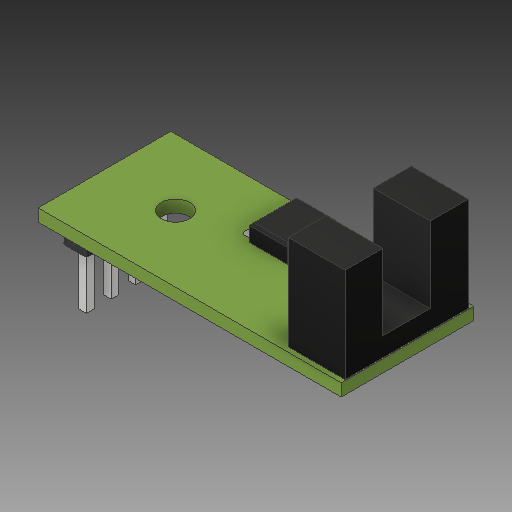
# Autodesk Inventor part: Оптический датчик
Saved by Autodesk Inventor 2019 (Build 230136000, 136)
## iProperties
Created: 2019-08-06
Part Number: Оптический датчик
Material: Типовые
Document SubType Name: Modeling
Designer: user
Density: 1 g/cm^3
Appearance: По умолчанию
Mass: 1.23373 g
Surface Area: 15.9477 cm^2
Volume: 1.23373 cm^3
Author: user
Autodesk Inventor part; units mm, degrees
ref_plane "YZ Plane" through (0, 0, 0) normal (1, 0, 0) x (0, 1, 0)
ref_plane "XZ Plane" through (0, 0, 0) normal (0, 1, 0) x (-1, 0, 0)
ref_plane "XY Plane" through (0, 0, 0) normal (0, 0, 1) x (1, 0, 0)
sketch "Эскиз1" plane through (0, 0, 0) normal (0, 1, 0) x (-1, 0, 0)
  line L0 (-16, 7) -> (16, 7)
  line L1 (16, 7) -> (16, -7)
  line L2 (16, -7) -> (-16, -7)
  line L3 (-16, -7) -> (-16, 7)
  line L4 (-16, 7) -> (16, -7) construction
  line L5 (16, 7) -> (-16, -7) construction
  point P0 (0, 0)
  dimension "d0" = 32
  dimension "d1" = 14
  constraints: 12 end point, 2 midpoint, 2 parallel, 1 horizontal, 1 perpendicular
  measures "d0" distance of L1.end L2.end
  measures "d1" distance of L0.end L1.end
extrude "Выдавливание1" add sketch "Эскиз1" along normal blind 1.3
sketch "Эскиз4" plane through (0, 1.3, 0) normal (0, 1, 0) x (1, 0, 0)
  line L0 (-16, -7) -> (16, -7) projected
  line L1 (16, -7) -> (16, -6.5)
  line L2 (16, -7) -> (16, 7) projected
  line L3 (16, -6.5) -> (15.9, -6.5)
  line L4 (15.9, -6.5) -> (9.9, -6.5)
  line L5 (9.9, -6.5) -> (9.9, 6.5)
  line L6 (9.9, 6.5) -> (15.9, 6.5)
  line L7 (15.9, 6.5) -> (15.9, -6.5)
  point P0 (0, 0)
  dimension "d13" = 0.5
  dimension "d14" = 0.1
  dimension "d15" = 6
  dimension "d16" = 13
  constraints: 12 end point, 2 parallel, 2 perpendicular, 1 horizontal, 1 point on line
  measures "d13" distance of L0.end L1.end
  measures "d14" distance of L1.end L3.end
  measures "d15" distance of L5.end L6.end
  measures "d16" distance of L4.end L5.end
extrude "Выдавливание4" add sketch "Эскиз4" along normal blind 10
sketch "Эскиз5" plane through (0, 11.3, 0) normal (0, 1, 0) x (1, 0, 0)
  line L0 (9.9, 6.5) -> (9.9, -6.5) projected
  line L1 (15.9, -2.5) -> (9.9, -2.5)
  line L2 (9.9, -2.5) -> (9.9, 2.5)
  line L3 (9.9, 2.5) -> (15.9, 2.5)
  line L4 (15.9, 2.5) -> (15.9, -2.5)
  line L5 (15.9, -2.5) -> (9.9, 2.5) construction
  line L6 (9.9, -2.5) -> (15.9, 2.5) construction
  point P0 (0, 0)
  point P1 (12.9, 0)
  dimension "d19" = 5
  constraints: 12 end point, 2 midpoint, 2 parallel, 1 horizontal, 1 perpendicular, 1 point on line
  measures "d19" distance of L1.end L2.end
extrude "Выдавливание5" cut sketch "Эскиз5" against normal blind 8
sketch "Эскиз6" plane through (0, 1.3, 0) normal (0, 1, 0) x (1, 0, 0)
  line L0 (-16, 7) -> (-16, -7) projected
  line L1 (-16, 0) -> (-10, 0)
  line L2 (-10, 0) -> (-7, 0)
  circle A0 centre (-8.5, 0) radius 1.5
  point P0 (0, 0)
  dimension "d22" = 6
  dimension "d23" = 3
  constraints: 4 end point, 2 midpoint, 1 horizontal, 1 horizontal alignment, 1 point on line, 2 other
  measures "d22" distance of L1.start L1.end
  measures "d23" distance of L1.end L2.end
extrude "Выдавливание6" cut sketch "Эскиз6" against normal blind 8
sketch "Эскиз10" plane through (0, 1.3, 0) normal (0, 1, 0) x (1, 0, 0)
  line L0 (2.3, 6) -> (-1.7, 6)
  line L1 (-1.7, 6) -> (-1.7, 1)
  line L2 (-1.7, 1) -> (2.3, 1)
  line L3 (2.3, 1) -> (2.3, 6)
  line L4 (-12.7, 2.9) -> (-12.7, 4.9) projected
  line L5 (16, 7) -> (-16, 7) projected
  point P0 (0, 0)
  dimension "d49" = 4
  dimension "d50" = 5
  dimension "d51" = 11
  dimension "d52" = 1
  constraints: 8 end point, 2 parallel, 1 horizontal, 1 perpendicular
  measures "d49" distance of L2.end L1.end
  measures "d50" distance of L1.end L0.end
  measures "d51" distance between parallel lines of L4 L1
  measures "d52" distance between parallel lines of L5 L0
extrude "Выдавливание9" add sketch "Эскиз10" along normal blind 1.8
chamfer "Фаска1" distance 0.25 angle 45 4 edges at (-1.7, 3.1, -3.5) (0.3, 3.1, -1) (2.3, 3.1, -3.5) (0.3, 3.1, -6)
sketch "Эскиз11" plane through (0, 1.3, 0) normal (0, 1, 0) x (1, 0, 0)
  line L0 (-1.7, 1) -> (-1.7, 6) projected
  line L1 (-1.7, 6) -> (-1.7, 5.8)
  line L2 (-1.7, 5.8) -> (-2.7, 5.8)
  line L3 (-2.7, 5.8) -> (-2.7, 5.3)
  line L4 (-2.7, 5.3) -> (-1.7, 5.3)
  line L5 (-1.7, 5.3) -> (-1.7, 5.8)
  line L6 (-1.7, 4.7) -> (-1.7, 4.5)
  line L7 (-1.7, 4.5) -> (-2.7, 4.5)
  line L8 (-2.7, 4.5) -> (-2.7, 4)
  line L9 (-2.7, 4) -> (-1.7, 4)
  line L10 (-1.7, 4) -> (-1.7, 4.5)
  line L11 (-1.7, 3.4) -> (-1.7, 3.2)
  line L12 (-1.7, 3.2) -> (-2.7, 3.2)
  line L13 (-2.7, 3.2) -> (-2.7, 2.7)
  line L14 (-2.7, 2.7) -> (-1.7, 2.7)
  line L15 (-1.7, 2.7) -> (-1.7, 3.2)
  line L16 (-1.7, 2.1) -> (-1.7, 1.9)
  line L17 (-1.7, 1.9) -> (-2.7, 1.9)
  line L18 (-2.7, 1.9) -> (-2.7, 1.4)
  line L19 (-2.7, 1.4) -> (-1.7, 1.4)
  line L20 (-1.7, 1.4) -> (-1.7, 1.9)
  line L21 (-1.7, 6) -> (2.3, 6) projected
  line L22 (0.3, 6) -> (0.3, 4.6)
  line L23 (2.3, 1) -> (2.3, 6)
  line L24 (2.3, 6) -> (2.3, 5.8)
  line L25 (2.3, 5.8) -> (3.3, 5.8)
  line L26 (3.3, 5.8) -> (3.3, 5.3)
  line L27 (3.3, 5.3) -> (2.3, 5.3)
  line L28 (2.3, 5.3) -> (2.3, 5.8)
  line L29 (2.3, 4.7) -> (2.3, 4.5)
  line L30 (2.3, 4.5) -> (3.3, 4.5)
  line L31 (3.3, 4.5) -> (3.3, 4)
  line L32 (3.3, 4) -> (2.3, 4)
  line L33 (2.3, 4) -> (2.3, 4.5)
  line L34 (2.3, 3.4) -> (2.3, 3.2)
  line L35 (2.3, 3.2) -> (3.3, 3.2)
  line L36 (3.3, 3.2) -> (3.3, 2.7)
  line L37 (3.3, 2.7) -> (2.3, 2.7)
  line L38 (2.3, 2.7) -> (2.3, 3.2)
  line L39 (2.3, 2.1) -> (2.3, 1.9)
  line L40 (2.3, 1.9) -> (3.3, 1.9)
  line L41 (3.3, 1.9) -> (3.3, 1.4)
  line L42 (3.3, 1.4) -> (2.3, 1.4)
  line L43 (2.3, 1.4) -> (2.3, 1.9)
  point P0 (0, 0)
  dimension "d58" = 0.2
  dimension "d59" = 1
  dimension "d60" = 0.5
  dimension "d63" = 1.3
  constraints: 84 end point, 20 symmetric about line, 2 parallel, 2 point on line, 2 vertical, 1 horizontal, 1 midpoint, 1 perpendicular, 30 other
  measures "d58" distance of L0.end L1.end
  measures "d59" distance of L4.end L3.end
  measures "d60" distance of L3.end L2.end
  measures "d63" distance of L1.end L6.end
extrude "Выдавливание10" add sketch "Эскиз11" along normal blind 1
chamfer "Фаска2" distance 0.75 angle 45 8 edges at (-2.7, 2.3, -5.55) (-2.7, 2.3, -4.25) (-2.7, 2.3, -2.95) (-2.7, 2.3, -1.65) (3.3, 2.3, -1.65) (3.3, 2.3, -2.95) (3.3, 2.3, -4.25) (3.3, 2.3, -5.55)
sketch "Эскиз18" plane through (0, 0, 0) normal (0, -1, 0) x (1, 0, 0)
  line L0 (16, 7) -> (-16, 7) projected
  line L1 (-16, 7) -> (-15.3, 7)
  line L2 (-15.3, 7) -> (-15.3, 5.2)
  line L3 (-15, 5.2) -> (-13, 5.2)
  line L4 (-12.7, 4.9) -> (-12.7, 2.9)
  line L5 (-13, 2.6) -> (-15, 2.6)
  line L6 (-15.3, 2.9) -> (-15.3, 4.9)
  arc A0 (-12.7, 4.9) -> (-13, 5.2) centre (-13, 4.9) ccw
  arc A1 (-13, 2.6) -> (-12.7, 2.9) centre (-13, 2.9) ccw
  arc A2 (-15.3, 2.9) -> (-15, 2.6) centre (-15, 2.9) ccw
  arc A3 (-15, 5.2) -> (-15.3, 4.9) centre (-15, 4.9) ccw
  line L7 (-15.3, 4.4) -> (-15.3, 2.6)
  arc A4 (-15, 2.6) -> (-15.3, 2.3) centre (-15, 2.3) ccw
  line L8 (-15, 2.6) -> (-13, 2.6)
  arc A5 (-12.7, 2.3) -> (-13, 2.6) centre (-13, 2.3) ccw
  line L9 (-15.3, 0.3) -> (-15.3, 2.3)
  arc A6 (-15.3, 0.3) -> (-15, 0) centre (-15, 0.3) ccw
  line L10 (-12.7, 2.3) -> (-12.7, 0.3)
  arc A7 (-13, 0) -> (-12.7, 0.3) centre (-13, 0.3) ccw
  line L11 (-13, 0) -> (-15, 0)
  line L12 (-15.3, 1.8) -> (-15.3, 0)
  arc A8 (-15, 0) -> (-15.3, -0.3) centre (-15, -0.3) ccw
  line L13 (-15, 0) -> (-13, 0)
  arc A9 (-12.7, -0.3) -> (-13, 0) centre (-13, -0.3) ccw
  line L14 (-15.3, -2.3) -> (-15.3, -0.3)
  arc A10 (-15.3, -2.3) -> (-15, -2.6) centre (-15, -2.3) ccw
  line L15 (-12.7, -0.3) -> (-12.7, -2.3)
  arc A11 (-13, -2.6) -> (-12.7, -2.3) centre (-13, -2.3) ccw
  line L16 (-13, -2.6) -> (-15, -2.6)
  line L17 (-15.3, -0.8) -> (-15.3, -2.6)
  arc A12 (-15, -2.6) -> (-15.3, -2.9) centre (-15, -2.9) ccw
  line L18 (-15, -2.6) -> (-13, -2.6)
  arc A13 (-12.7, -2.9) -> (-13, -2.6) centre (-13, -2.9) ccw
  line L19 (-15.3, -4.9) -> (-15.3, -2.9)
  arc A14 (-15.3, -4.9) -> (-15, -5.2) centre (-15, -4.9) ccw
  line L20 (-12.7, -2.9) -> (-12.7, -4.9)
  arc A15 (-13, -5.2) -> (-12.7, -4.9) centre (-13, -4.9) ccw
  line L21 (-13, -5.2) -> (-15, -5.2)
  point P0 (0, 0)
  point P1 (-12.7, 2.6)
  point P2 (-12.7, 5.2)
  point P3 (-12.7, 2.6)
  point P4 (-12.7, 0)
  point P5 (-12.7, 0)
  point P6 (-12.7, -2.6)
  point P7 (-12.7, -2.6)
  point P8 (-15.3, -5.2)
  point P9 (-12.7, -5.2)
  dimension "d105" = 0.7
  dimension "d106" = 1.8
  dimension "d107" = 2.6
  dimension "d108" = 2.6
  dimension "d109" = 0.3
  dimension "d112" = 2.6
  constraints: 42 end point, 33 point on line, 32 point on circle, 16 centre point, 8 tangent, 3 equal radius, 2 parallel, 2 vertical, 1 collinear, 1 horizontal, 1 perpendicular, 77 other
  measures "d105" distance of L0.end L1.end
  measures "d106" distance of L1.end L2.end
  measures "d107" distance of point (-12.7, 2.6) point (-15.3, 2.6)
  measures "d108" distance of point (-12.7, 5.2) point (-12.7, 2.6)
  measures "d109" radius of A0
  measures "d112" distance of L6.start L9.start
extrude "Выдавливание11" add sketch "Эскиз18" along normal blind 2.5
sketch "Эскиз19" plane through (0, -2.5, 0) normal (0, -1, 0) x (1, 0, 0)
  line L0 (-15, 5.2) -> (-13, 5.2) projected
  line L1 (-14, 5.2) -> (-14, 3.9)
  line L2 (-14.4, 3.5) -> (-13.6, 3.5)
  line L3 (-13.6, 3.5) -> (-13.6, 4.3)
  line L4 (-13.6, 4.3) -> (-14.4, 4.3)
  line L5 (-14.4, 4.3) -> (-14.4, 3.5)
  line L6 (-14.4, 3.5) -> (-13.6, 4.3) construction
  line L7 (-13.6, 3.5) -> (-14.4, 4.3) construction
  line L8 (-14.4, 0.9) -> (-13.6, 0.9)
  line L9 (-13.6, 0.9) -> (-13.6, 1.7)
  line L10 (-13.6, 1.7) -> (-14.4, 1.7)
  line L11 (-14.4, 1.7) -> (-14.4, 0.9)
  line L12 (-14.4, 0.9) -> (-13.6, 1.7) construction
  line L13 (-13.6, 0.9) -> (-14.4, 1.7) construction
  line L14 (-14.4, -1.7) -> (-13.6, -1.7)
  line L15 (-13.6, -1.7) -> (-13.6, -0.9)
  line L16 (-13.6, -0.9) -> (-14.4, -0.9)
  line L17 (-14.4, -0.9) -> (-14.4, -1.7)
  line L18 (-14.4, -1.7) -> (-13.6, -0.9) construction
  line L19 (-13.6, -1.7) -> (-14.4, -0.9) construction
  line L20 (-14.4, -4.3) -> (-13.6, -4.3)
  line L21 (-13.6, -4.3) -> (-13.6, -3.5)
  line L22 (-13.6, -3.5) -> (-14.4, -3.5)
  line L23 (-14.4, -3.5) -> (-14.4, -4.3)
  line L24 (-14.4, -4.3) -> (-13.6, -3.5) construction
  line L25 (-13.6, -4.3) -> (-14.4, -3.5) construction
  point P0 (0, 0)
  point P1 (-14, 1.3)
  point P2 (-14, -1.3)
  point P3 (-14, -3.9)
  dimension "d119" = 1.3
  dimension "d120" = 0.8
  dimension "d121" = 0.8
  dimension "d124" = 2.6
  constraints: 50 end point, 9 midpoint, 2 parallel, 2 vertical, 1 horizontal, 1 perpendicular, 33 other
  measures "d119" distance of L1.start L1.end
  measures "d120" distance of L4.end L3.end
  measures "d121" distance of L3.end L2.end
  measures "d124" distance of L1.end point (-14, 1.3)
extrude "Выдавливание12" add sketch "Эскиз19" along normal blind 6
